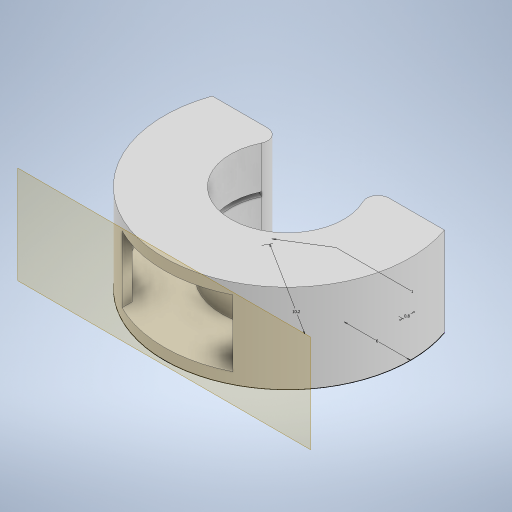
# Autodesk Inventor part: ir다이오드3
Saved by Autodesk Inventor 2023 (Build 270158000, 158)
## iProperties
Created: 2023-04-25
Part Number: ir다이오드3
Material: 일반
Document SubType Name: Modeling
Designer: rlatk
Density: 1 g/cm^3
Appearance: 기본값
Author: rlatk
Autodesk Inventor part; units mm, degrees
ref_plane "YZ Plane" through (0, 0, 0) normal (1, 0, 0) x (0, 1, 0)
ref_plane "XZ Plane" through (0, 0, 0) normal (0, 1, 0) x (-1, 0, 0)
ref_plane "XY Plane" through (0, 0, 0) normal (0, 0, 1) x (1, 0, 0)
sketch "스케치1" plane through (0, 0, 0) normal (0, 1, 0) x (-1, 0, 0)
  arc A0 (4.5746, -2.2545) -> (-4.5746, -2.2545) centre (0, 0) ccw
  arc A1 (10.4664, -3.6965) -> (-10.4664, -3.6965) centre (0, 0) ccw
  line L0 (10.4664, -3.6965) -> (5.4716, -3.6965)
  line L1 (-5.4716, -3.6965) -> (-10.4664, -3.6965)
  arc A2 (4.5746, -2.2545) -> (5.4716, -3.6965) centre (5.4716, -2.6965) ccw
  arc A3 (-5.4716, -3.6965) -> (-4.5746, -2.2545) centre (-5.4716, -2.6965) ccw
  arc A4 (9.8843, -2.8965) -> (-9.8843, -2.8965) centre (0, 0) ccw
  line L2 (9.8843, -2.8965) -> (5.4716, -2.8965)
  arc A5 (5.2922, -2.6081) -> (5.4716, -2.8965) centre (5.4716, -2.6965) ccw
  arc A6 (5.2922, -2.6081) -> (-5.2922, -2.6081) centre (0, 0) ccw
  arc A7 (-5.4716, -2.8965) -> (-5.2922, -2.6081) centre (-5.4716, -2.6965) ccw
  line L3 (-5.4716, -2.8965) -> (-9.8843, -2.8965)
  line L4 (-5.2922, -2.6081) -> (-4.5746, -2.2545)
  line L5 (5.2922, -2.6081) -> (4.5746, -2.2545)
  point P0 (-3.5136, -3.6965)
  point P1 (3.5136, -3.6965)
  dimension "d0" = 10.2
  dimension "d1" = 6
  dimension "d2" = 1
  dimension "d5" = 0.8
  constraints: 18 point on circle, 12 end point, 8 centre point, 4 tangent, 2 horizontal, 2 point on line, 1 coincident, 1 equal radius, 5 other
  measures "d0" diameter of A0
  measures "d1" radial gap between concentric circles of A0 A1
  measures "d2" radius of A2
  measures "d5" distance between parallel lines of L1 L3
extrude "돌출7" add sketch "스케치1" along normal blind 8
extrude "돌출8" cut sketch "스케치1" along normal blind 7 contours A6 A7 L3 A4 L2 A5
extrude "돌출9" add sketch "스케치1" along normal blind 1 contours A6 A7 L3 A4 L2 A5
extrude "돌출10" cut sketch "스케치1" along normal blind 4.2 contours A0 L4 A6 L5
extrude "돌출11" add sketch "스케치1" along normal blind 3.8 contours A0 L4 A6 L5
ref_plane "작업 평면2" through (0, 0, 11.1) normal (0, 0, 1) x (1, 0, 0)
sketch "스케치4" plane through (0, 0, 11.1) normal (0, 0, 1) x (1, 0, 0)
  line L0 (10.3, 7) -> (-10.3, 7) projected
  line L1 (-10.3, 1) -> (10.3, 1) projected
  line L2 (10.3, 1) -> (10.3, 7) projected
  line L3 (-10.3, 1) -> (-10.3, 7) projected
  line L4 (11.1, 8) -> (-11.1, 8) projected
  line L5 (11.1, 0) -> (-11.1, 0) projected
  line L6 (0, 7) -> (5, 7)
  line L7 (5, 7) -> (5, 1)
  line L8 (5, 1) -> (0, 1)
  line L9 (0, 7) -> (-5, 7)
  line L10 (-5, 7) -> (-5, 1)
  line L11 (-5, 1) -> (0, 1)
  line L12 (0, 8) -> (0, 7)
  line L13 (0, 1) -> (0, 0)
  point P0 (-9.8843, 7)
  point P1 (9.8843, 7)
  point P2 (9.8843, 1)
  point P3 (-9.8843, 1)
  point P4 (-10.4664, 8)
  point P5 (10.4664, 8)
  point P6 (-10.4664, 0)
  point P7 (10.4664, 0)
  dimension "d27" = 5
  constraints: 16 end point, 3 midpoint, 3 perpendicular, 2 point on line
  measures "d27" distance of L6.start L6.end
extrude "돌출12" cut sketch "스케치4" against normal blind 3.8 contours L7 L1 L10 L0
